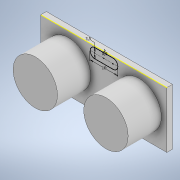
# Autodesk Inventor part: Ultrasonic HC-SRO4
Saved by Autodesk Inventor 2020 (Build 240168000, 168)
## iProperties
Created: 2021-04-26
Part Number: Ultrasonic HC-SRO4
Material: Типовые
Document SubType Name: Modeling
Designer: Антон
Density: 1 g/cm^3
Appearance: По умолчанию
Author: Антон
Autodesk Inventor part; units mm, degrees
ref_plane "YZ Plane" through (0, 0, 0) normal (1, 0, 0) x (0, 1, 0)
ref_plane "XZ Plane" through (0, 0, 0) normal (0, 1, 0) x (-1, 0, 0)
ref_plane "XY Plane" through (0, 0, 0) normal (0, 0, 1) x (1, 0, 0)
sketch "Эскиз1" plane through (0, 0, 0) normal (0, 0, 1) x (1, 0, 0)
  line L0 (0, 0) -> (45.5, 0)
  line L1 (45.5, 0) -> (45.5, 20.3)
  line L2 (45.5, 20.3) -> (0, 20.3)
  line L3 (0, 20.3) -> (0, 0)
  dimension "d0" = 45.5
  dimension "d1" = 20.3
  constraints: 8 end point, 2 parallel, 1 horizontal, 1 perpendicular
  measures "d0" distance of L2.end L1.end
  measures "d1" distance of L1.end L0.end
extrude "Выдавливание1" add sketch "Эскиз1" along normal blind 2
sketch "Эскиз2" plane through (0, 0, 2) normal (0, 0, 1) x (1, 0, 0)
  line L0 (0, 20.3) -> (0, 0) projected
  line L1 (0, 10.15) -> (2, 10.15)
  line L2 (2, 10.15) -> (10, 10.15)
  circle A0 centre (10, 10.15) radius 8
  line L3 (45.5, 20.3) -> (0, 20.3) projected
  line L4 (22.75, 20.3) -> (22.75, 0)
  line L5 (0, 0) -> (45.5, 0) projected
  circle A1 centre (35.5, 10.15) radius 8
  dimension "d5" = 16
  dimension "d4" = 2
  constraints: 6 end point, 3 midpoint, 2 horizontal, 1 centre point, 1 coincident, 1 horizontal alignment, 1 symmetric about line, 3 other
  measures "d4" distance of L1.start L1.end
extrude "Выдавливание2" add sketch "Эскиз2" along normal blind 12 contours A0 | A1
sketch "Эскиз3" plane through (0, 0, 2) normal (0, 0, 1) x (1, 0, 0)
  line L0 (45.5, 20.3) -> (0, 20.3) projected
  line L1 (22.75, 20.3) -> (22.75, 19.8)
  line L2 (27.75, 18.05) -> (17.75, 18.05) construction
  line L3 (26, 19.8) -> (19.5, 19.8)
  line L4 (19.5, 16.3) -> (26, 16.3)
  arc A0 (26, 16.3) -> (26, 19.8) centre (26, 18.05) ccw
  arc A1 (19.5, 19.8) -> (19.5, 16.3) centre (19.5, 18.05) ccw
  point P0 (0, 0)
  point P1 (22.75, 18.05)
  dimension "d8" = 0.5
  dimension "d9" = 10
  dimension "d10" = 3.5
  constraints: 10 end point, 6 point on circle, 4 tangent, 3 midpoint, 2 centre point, 2 point on line, 1 horizontal, 1 parallel, 1 vertical
  measures "d8" distance of L1.end L1.start
  measures "d9" distance of L2.start L2.end
  measures "d10" diameter of A1
